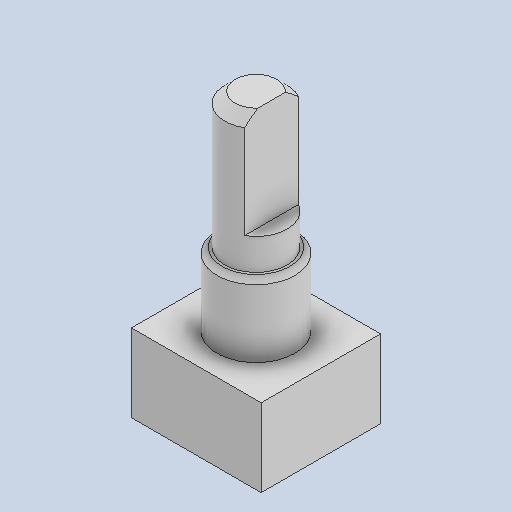
# Autodesk Inventor part: rotery
Saved by Autodesk Inventor 2025.2 (Build 292293000, 293)
## iProperties
Created: 2025-04-09
Part Number: rotery
Material: Generic
Document SubType Name: Modeling
Designer: mirewn
Density: 1 g/cm^3
Appearance: Default
Author: mirewn
Autodesk Inventor part; units mm, degrees
ref_plane "YZ Plane" through (0, 0, 0) normal (1, 0, 0) x (0, 1, 0)
ref_plane "XZ Plane" through (0, 0, 0) normal (0, 1, 0) x (-1, 0, 0)
ref_plane "XY Plane" through (0, 0, 0) normal (0, 0, 1) x (1, 0, 0)
sketch "Sketch1" plane through (0, 0, 0) normal (0, 1, 0) x (-1, 0, 0)
  line L0 (6.25, 5.75) -> (-6.25, 5.75)
  line L1 (-6.25, 5.75) -> (-6.25, -5.75)
  line L2 (-6.25, -5.75) -> (6.25, -5.75)
  line L3 (6.25, -5.75) -> (6.25, 5.75)
  line L4 (6.25, 5.75) -> (-6.25, -5.75) construction
  line L5 (-6.25, 5.75) -> (6.25, -5.75) construction
  point P0 (0, 0)
  dimension "d0" = 12.5
  dimension "d1" = 11.5
  constraints: 12 end point, 2 midpoint, 2 parallel, 1 horizontal, 1 perpendicular
  measures "d0" distance of L2.end L1.end
  measures "d1" distance between parallel lines of L2 L0
extrude "Extrusion1" add sketch "Sketch1" along normal blind 7.5
sketch "Sketch2" plane through (0, 7.5, 0) normal (0, 1, 0) x (1, 0, 0)
  circle A0 centre (0, 0) radius 3.75
  dimension "d4" = 7.5
  constraints: 1 centre point, 1 coincident
  measures "d4" diameter of A0
extrude "Extrusion2" add sketch "Sketch2" along normal blind 7
sketch "Sketch3" plane through (0, 14.5, 0) normal (0, 1, 0) x (1, 0, 0)
  circle A0 centre (0, 0) radius 3
  dimension "d7" = 6
  constraints: 1 centre point, 1 coincident
  measures "d7" diameter of A0
extrude "Extrusion3" add sketch "Sketch3" along normal blind 13
sketch "Sketch4" plane through (0, 27.5, 0) normal (0, 1, 0) x (1, 0, 0)
  circle A0 centre (0, 0) radius 3 projected
  line L0 (1.5, -2.5981) -> (1.5, 2.5981)
  line L1 (3, 0) -> (-9, 0) construction
  circle A1 centre (0, 0) radius 3.75 construction
  circle A2 centre (0, 0) radius 3 construction
  point P0 (-3, 0)
  dimension "d10" = 4.5
  constraints: 4 end point, 4 point on circle, 1 coincident, 1 midpoint, 1 perpendicular, 1 vertical, 3 other
  measures "d10" distance from line of L0 point (-3, 0)
extrude "Extrusion4" cut sketch "Sketch4" against normal blind 10 contours A0 L0 picked at (1.6691, 0.7431)
chamfer "Chamfer1" distance 0.5 angle 45 1 edges at (-3.75, 14.5, 0)
chamfer "Chamfer2" distance 1 angle 45 1 edges at (-3, 27.5, 0)
body "Solid1"
